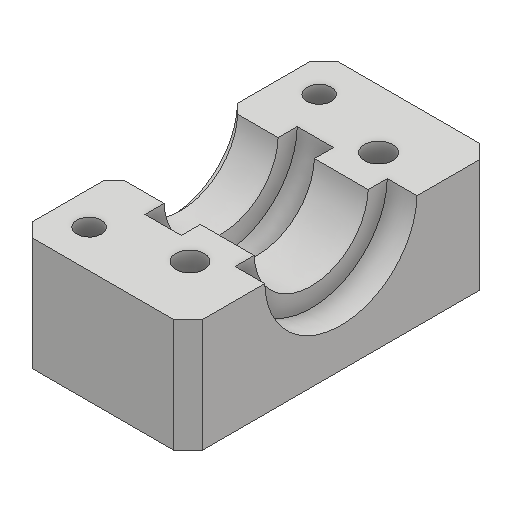
# Autodesk Inventor part: 3DP_ABS_E3D_V6_Mount_Clamp
Saved by Autodesk Inventor 2026.1 (Build 301233000, 233)
## iProperties
Created: 2016-06-18
Part Number: 3DP_ABS_E3D_V6_Mount_Clamp
Material: Ogólny
Document SubType Name: Modeling
Designer: Andrzej
Density: 1 g/cm^3
Appearance: Domyślna
Mass: 4.78775 g
Surface Area: 24.3351 cm^2
Volume: 4.78775 cm^3
Author: Andrzej
Autodesk Inventor part; units mm, degrees
ref_plane "YZ Plane" through (0, 0, 0) normal (1, 0, 0) x (0, 1, 0)
ref_plane "XZ Plane" through (0, 0, 0) normal (0, 1, 0) x (-1, 0, 0)
ref_plane "XY Plane" through (0, 0, 0) normal (0, 0, 1) x (1, 0, 0)
sketch "Szkic1" plane through (0, 0, 0) normal (0, 0, 1) x (1, 0, 0)
  line L0 (-10.699, 18.8462) -> (5.301, 18.8462)
  line L1 (5.301, 18.8462) -> (5.301, -13.5538)
  line L2 (5.301, -13.5538) -> (-10.699, -13.5538)
  line L3 (-10.699, -13.5538) -> (-10.699, 18.8462)
  point P0 (0, 0)
  dimension "d0" = 16
  dimension "d1" = 32.4
  constraints: 8 end point, 2 parallel, 1 horizontal, 1 perpendicular
  measures "d0" distance of L1.end L2.end
  measures "d1" distance of L0.end L1.end
extrude "Wyciągnięcie proste1" add sketch "Szkic1" along normal blind 12
sketch "Szkic2" plane through (-10.699, -13.5538, 0) normal (-1, 0, 0) x (0, 0, 1)
  line L0 (0, 0) -> (0, 32.4) projected
  line L1 (0, 0) -> (12, 0) projected
  line L2 (12, 32.4) -> (12, 0) projected
  line L3 (0, 32.4) -> (12, 32.4) projected
  line L4 (12, 32.4) -> (12, 0) projected
  circle A0 centre (12.2, 16.2) radius 6.05
  point P0 (0, 13.5538)
  dimension "d4" = 32.4
  dimension "d6" = 12.1
  dimension "d66" = 16.2
  dimension "d67" = 0.2
  constraints: 1 centre point
  measures "d4" distance of L2.start L1.end
  measures "d6" diameter of A0
  measures "d66" distance from line of L3 A0.centre
  measures "d67" distance from line of L2 A0.centre
extrude "Wyciągnięcie proste2" cut sketch "Szkic2" against normal blind 13 contours A0 L2 | L2 A0
sketch "Szkic3" plane through (-10.699, -13.5538, 0) normal (-1, 0, 0) x (0, 0, 1)
  arc A0 (12, 22.2467) -> (12, 10.1533) centre (12.2, 16.2) ccw projected
  line L0 (12, 32.4) -> (12, 22.2467) projected
  line L1 (0, 32.4) -> (12, 32.4) projected
  line L2 (0, 0) -> (0, 32.4) projected
  line L3 (0, 0) -> (12, 0) projected
  line L4 (12, 10.1533) -> (12, 0) projected
  arc A1 (12, 24.2725) -> (12, 8.1275) centre (12.2, 16.2) ccw
  point P0 (0, 13.5538)
  dimension "d9" = 16.15
  constraints: 2 point on circle, 2 point on line, 1 centre point, 1 coincident
  measures "d9" diameter of A1
extrude "Wyciągnięcie proste3" cut sketch "Szkic3" against normal blind 7.15 contours A0 L4 A1 L0
extrude "Wyciągnięcie proste4" add sketch "Szkic3" against normal blind 3.3 contours A0 L4 A1 L0
sketch "Szkic6" plane through (5.301, -13.5538, 0) normal (1, 0, 0) x (0, 0, -1)
  arc A0 (-12, 8.1275) -> (-12, 24.2725) centre (-12.2, 16.2) ccw projected
  line L0 (0, 32.4) -> (0, 0) projected
  line L1 (0, 32.4) -> (-12, 32.4) projected
  line L2 (-12, 0) -> (-12, 32.4) projected
  line L3 (0, 0) -> (-12, 0) projected
  arc A1 (-12, 8.1275) -> (-12, 24.2725) centre (-12.2, 16.2) ccw
  point P0 (0, 13.5538)
  constraints: 2 point on circle, 2 point on line, 1 centre point, 1 coincident, 1 concentric
extrude "Wyciągnięcie proste5" cut sketch "Szkic6" against normal blind 3.15 contours L2 A0
sketch "Szkic7" plane through (0, 0, 12) normal (0, 0, 1) x (1, 0, 0)
  line L0 (5.301, -5.4264) -> (2.151, -5.4264) projected
  line L1 (2.151, -5.4264) -> (2.151, -3.4005) projected
  line L2 (2.151, -3.4005) -> (-3.549, -3.4005) projected
  line L3 (-3.549, -3.4005) -> (-3.549, -5.4264) projected
  line L4 (-3.549, -5.4264) -> (-7.399, -5.4264) projected
  line L5 (-7.399, -3.4005) -> (-7.399, -5.4264) projected
  line L6 (-10.699, -3.4005) -> (-7.399, -3.4005) projected
  line L7 (-10.699, -3.4005) -> (-10.699, -13.5538) projected
  line L8 (-10.699, -13.5538) -> (5.301, -13.5538) projected
  line L9 (5.301, -13.5538) -> (5.301, -5.4264) projected
  line L10 (2.151, 10.7187) -> (5.301, 10.7187) projected
  line L11 (5.301, 10.7187) -> (5.301, 18.8462) projected
  line L12 (5.301, 18.8462) -> (-10.699, 18.8462) projected
  line L13 (-10.699, 18.8462) -> (-10.699, 8.6929) projected
  line L14 (-10.699, 8.6929) -> (-7.399, 8.6929) projected
  line L15 (-7.399, 10.7187) -> (-7.399, 8.6929) projected
  line L16 (-7.399, 10.7187) -> (-3.549, 10.7187) projected
  line L17 (-3.549, 10.7187) -> (-3.549, 8.6929) projected
  line L18 (-3.549, 8.6929) -> (2.151, 8.6929) projected
  line L19 (2.151, 8.6929) -> (2.151, 10.7187) projected
  point P0 (0, 0)
  point P1 (-0.699, -7.3538)
  point P2 (-0.699, 12.6462)
  dimension "d46" = 20
  dimension "d47" = 32.4
  dimension "d48" = 6.2
  dimension "d49" = 6.2
  dimension "d50" = 5.7
  dimension "d68" = 10
  dimension "d69" = 10
  measures "d46" distance of point (-0.699, 12.646) point (-0.699, -7.354)
  measures "d47" distance between parallel lines of L12 L8
  measures "d48" distance from line of L8 point (-0.699, -7.354)
  measures "d49" distance from line of L12 point (-0.699, 12.646)
  measures "d50" distance between parallel lines of L1 L3
  measures "d68" distance from line of L7 point (-0.699, -7.354)
  measures "d69" distance from line of L13 point (-0.699, 12.646)
hole "Otwór3" at (-0.699, -7.3538, 12) at (-0.699, 12.6462, 12) direction (0, 0, -1) diameter 3 end through all
sketch "Szkic8" plane through (-10.699, -13.5538, 0) normal (-1, 0, 0) x (0, 0, 1)
  line L0 (12, 32.4) -> (12, 22.2467) projected
  line L1 (0, 32.4) -> (12, 32.4) projected
  line L2 (0, 0) -> (0, 32.4) projected
  line L3 (0, 0) -> (12, 0) projected
  line L4 (12, 10.1533) -> (12, 0) projected
  arc A0 (12, 22.2467) -> (12, 10.1533) centre (12.2, 16.2) ccw projected
  point P0 (0, 13.5538)
extrude "Wyciągnięcie proste6" add sketch "Szkic8" along normal blind 2
chamfer "Faza4" distance 1 angle 45 1 edges at (-12.699, 2.6462, 6.15)
chamfer "Faza5" distance 1.5 angle 45 4 edges at (-12.699, 18.8462, 6) (5.301, 18.8462, 6) (-12.699, -13.5538, 6) (5.301, -13.5538, 6)
sketch "Szkic9" plane through (0, 0, 12) normal (0, 0, 1) x (1, 0, 0)
  line L0 (5.301, -12.0538) -> (3.801, -13.5538) projected
  line L1 (5.301, -12.0538) -> (5.301, -5.4264) projected
  line L2 (5.301, -5.4264) -> (2.151, -5.4264) projected
  line L3 (2.151, -5.4264) -> (2.151, -3.4005) projected
  line L4 (2.151, -3.4005) -> (-3.549, -3.4005) projected
  line L5 (-3.549, -3.4005) -> (-3.549, -5.4264) projected
  line L6 (-3.549, -5.4264) -> (-7.399, -5.4264) projected
  line L7 (-7.399, -3.4005) -> (-7.399, -5.4264) projected
  line L8 (-11.699, -3.4005) -> (-7.399, -3.4005) projected
  line L9 (-12.699, -12.0538) -> (-12.699, -4.401) projected
  line L10 (-11.199, -13.5538) -> (-12.699, -12.0538) projected
  line L11 (3.801, -13.5538) -> (-11.199, -13.5538) projected
  circle A0 centre (-0.699, -7.3538) radius 1.5 projected
  line L12 (3.801, 18.8462) -> (5.301, 17.3462) projected
  line L13 (3.801, 18.8462) -> (-11.199, 18.8462) projected
  line L14 (-12.699, 17.3462) -> (-11.199, 18.8462) projected
  line L15 (-12.699, 9.6933) -> (-12.699, 17.3462) projected
  line L16 (-7.399, 8.6929) -> (-11.699, 8.6929) projected
  line L17 (-7.399, 10.7187) -> (-7.399, 8.6929) projected
  line L18 (-7.399, 10.7187) -> (-3.549, 10.7187) projected
  line L19 (-3.549, 10.7187) -> (-3.549, 8.6929) projected
  line L20 (-3.549, 8.6929) -> (2.151, 8.6929) projected
  line L21 (2.151, 8.6929) -> (2.151, 10.7187) projected
  line L22 (2.151, 10.7187) -> (5.301, 10.7187) projected
  line L23 (5.301, 10.7187) -> (5.301, 17.3462) projected
  circle A1 centre (-0.699, 12.6462) radius 1.5 projected
  point P0 (0, 0)
  point P1 (-9.199, -9.5538)
  point P2 (-9.199, 14.8462)
  dimension "d78" = 3.5
  dimension "d79" = 3.5
  dimension "d80" = 4
  dimension "d81" = 4
  constraints: 2 other
  measures "d78" distance from line of L9 point (-9.199, -9.554)
  measures "d79" distance from line of L15 point (-9.199, 14.846)
  measures "d80" distance from line of L11 point (-9.199, -9.554)
  measures "d81" distance from line of L13 point (-9.199, 14.846)
hole "Otwór4" at (-9.199, -9.5538, 12) at (-9.199, 14.8462, 12) direction (0, 0, -1) diameter 2.6 end through all
equation "\"d48\" = -0.5 * d46 + 0.5 * d47"
